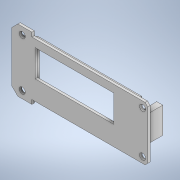
# Autodesk Inventor part: Деталь56
Saved by Autodesk Inventor 2020 (Build 240168000, 168)
## iProperties
Created: 2022-03-19
Part Number: Деталь56
Material: Типовые
Document SubType Name: Modeling
Designer: NoName
Density: 1 g/cm^3
Appearance: По умолчанию
Author: NoName
Autodesk Inventor part; units mm, degrees
ref_plane "YZ Plane" through (0, 0, 0) normal (1, 0, 0) x (0, 1, 0)
ref_plane "XZ Plane" through (0, 0, 0) normal (0, 1, 0) x (-1, 0, 0)
ref_plane "XY Plane" through (0, 0, 0) normal (0, 0, 1) x (1, 0, 0)
sketch "Эскиз1" plane through (0, 0, 0) normal (0, 0, 1) x (1, 0, 0)
  line L0 (40.25, 0.65) -> (37.25, 0.65) projected
  line L1 (37.25, 0.65) -> (37.25, -2.2) projected
  arc A0 (37.25, -2.2) -> (39.25, -4.2) centre (39.25, -2.2) ccw projected
  line L2 (39.25, -4.2) -> (39.25, -12.9) projected
  arc A1 (39.25, -12.9) -> (37.25, -14.9) centre (39.25, -14.9) ccw projected
  line L3 (37.25, -14.9) -> (37.25, -17.75) projected
  line L4 (37.25, -17.75) -> (40.25, -17.75) projected
  line L5 (40.25, -17.75) -> (41.25, -16.75) projected
  line L6 (41.25, -16.75) -> (41.25, -0.35) projected
  line L7 (41.25, -0.35) -> (40.25, 0.65) projected
  circle A2 centre (39.3375, -15.55) radius 1 projected
  circle A3 centre (39.3375, -1.55) radius 1 projected
  line L8 (2.55, -18.95) -> (2.55, -17.75) projected
  line L9 (2.55, -17.75) -> (2.55, -16.45) projected
  line L10 (0.65, -14.55) -> (2.55, -16.45) projected
  line L11 (-4.15, -14.55) -> (0.65, -14.55) projected
  line L12 (-4.15, -14.55) -> (-4.15, -16.95) projected
  line L13 (-4.15, -16.95) -> (-2.15, -18.95) projected
  line L14 (-2.15, -18.95) -> (2.55, -18.95) projected
  circle A4 centre (-0.65, -16.55) radius 1 projected
  line L15 (2.55, 0.65) -> (2.55, 1.85) projected
  line L16 (2.55, 1.85) -> (-2.15, 1.85) projected
  line L17 (-2.15, 1.85) -> (-4.15, -0.15) projected
  line L18 (-4.15, -0.15) -> (-4.15, -2.55) projected
  line L19 (0.65, -2.55) -> (-4.15, -2.55) projected
  line L20 (2.55, -0.65) -> (0.65, -2.55) projected
  line L21 (2.55, -0.65) -> (2.55, 0.65) projected
  circle A5 centre (-0.65, -0.55) radius 1 projected
  line L22 (2.55, 0.65) -> (40.25, 0.65) projected
  line L23 (40.25, -17.75) -> (2.55, -17.75) projected
  line L24 (-4.15, -14.55) -> (-4.15, -2.55) projected
  point P0 (0, 0)
extrude "Выдавливание1" add sketch "Эскиз1" along normal blind 0.8
sketch "Эскиз2" plane through (0, 0, 0.8) normal (0, 0, 1) x (1, 0, 0)
  line L0 (3.65, -11.05) -> (29.75, -11.05)
  line L1 (29.75, -11.05) -> (29.75, -2.05)
  line L2 (29.75, -2.05) -> (3.65, -2.05)
  line L3 (3.65, -2.05) -> (3.65, -11.05)
  line L4 (40.25, 0.65) -> (2.55, 0.65) projected
  line L5 (41.25, -16.75) -> (41.25, -0.35) projected
  point P0 (0, 0)
  dimension "d2" = 9
  dimension "d3" = 26.1
  dimension "d4" = 2.7
  dimension "d5" = 11.5
  constraints: 8 end point, 2 parallel, 1 horizontal, 1 perpendicular
  measures "d2" distance between parallel lines of L0 L2
  measures "d3" distance between parallel lines of L1 L3
  measures "d4" distance between parallel lines of L4 L2
  measures "d5" distance between parallel lines of L5 L1
extrude "Выдавливание2" cut sketch "Эскиз2" against normal through all
sketch "Эскиз3" plane through (0, 0, 0) normal (0, 0, -1) x (-1, 0, 0)
  line L0 (-40.25, 0.65) -> (-37.25, 0.65) projected
  line L1 (-37.25, 0.65) -> (-37.25, -2.2) projected
  arc A0 (-39.25, -4.2) -> (-37.25, -2.2) centre (-39.25, -2.2) ccw projected
  line L2 (-39.25, -4.2) -> (-39.25, -12.9) projected
  arc A1 (-37.25, -14.9) -> (-39.25, -12.9) centre (-39.25, -14.9) ccw projected
  line L3 (-37.25, -14.9) -> (-37.25, -17.75) projected
  line L4 (-37.25, -17.75) -> (-40.25, -17.75) projected
  line L5 (-40.25, -17.75) -> (-41.25, -16.75) projected
  line L6 (-41.25, -16.75) -> (-41.25, -0.35) projected
  line L7 (-41.25, -0.35) -> (-40.25, 0.65) projected
  circle A2 centre (-39.3375, -15.55) radius 1 projected
  circle A3 centre (-39.3375, -1.55) radius 1 projected
  line L8 (-2.55, 0.65) -> (-2.55, 1.85) projected
  line L9 (-2.55, 1.85) -> (2.15, 1.85) projected
  line L10 (2.15, 1.85) -> (4.15, -0.15) projected
  line L11 (4.15, -0.15) -> (4.15, -2.55) projected
  line L12 (-0.65, -2.55) -> (4.15, -2.55) projected
  line L13 (-2.55, -0.65) -> (-0.65, -2.55) projected
  line L14 (-2.55, -0.65) -> (-2.55, 0.65) projected
  circle A4 centre (0.65, -0.55) radius 1 projected
  line L15 (-2.55, -18.95) -> (-2.55, -17.75) projected
  line L16 (-2.55, -17.75) -> (-2.55, -16.45) projected
  line L17 (-0.65, -14.55) -> (-2.55, -16.45) projected
  line L18 (4.15, -14.55) -> (-0.65, -14.55) projected
  line L19 (4.15, -14.55) -> (4.15, -16.95) projected
  line L20 (4.15, -16.95) -> (2.15, -18.95) projected
  line L21 (2.15, -18.95) -> (-2.55, -18.95) projected
  circle A5 centre (0.65, -16.55) radius 1 projected
  line L22 (-2.55, -17.75) -> (-40.25, -17.75) projected
  line L23 (4.15, -2.55) -> (4.15, -14.55)
  line L24 (4.15, -0.15) -> (4.15, -16.95) projected
  line L25 (-3.25, -13.35) -> (-35.75, -13.35)
  line L26 (-35.75, -13.35) -> (-35.75, -1.45)
  line L27 (-35.75, -1.45) -> (-3.25, -1.45)
  line L28 (-3.25, -1.45) -> (-3.25, -13.35)
  line L29 (-29.75, -11.05) -> (-29.75, -2.05) projected
  line L30 (-3.65, -11.05) -> (-29.75, -11.05) projected
  line L31 (-3.65, -2.05) -> (-3.65, -11.05) projected
  line L32 (-29.75, -2.05) -> (-3.65, -2.05) projected
  line L33 (2.15, 1.85) -> (-43.25, 1.85) projected
  line L34 (-43.25, -18.95) -> (2.15, -18.95) projected
  line L35 (-37.25, -0.15) -> (-2.55, -0.15)
  line L36 (-37.25, -16.95) -> (-2.55, -16.95)
  point P0 (0, 0)
  dimension "d13" = 6
  dimension "d15" = 0.4
  dimension "d17" = 2.3
  dimension "d18" = 0.6
  dimension "d21" = 2
  dimension "d22" = 2
  constraints: 14 end point, 4 point on line, 3 perpendicular, 2 parallel, 1 collinear, 1 horizontal
  measures "d13" distance between parallel lines of L26 L29
  measures "d15" distance between parallel lines of L31 L28
  measures "d17" distance between parallel lines of L25 L30
  measures "d18" distance between parallel lines of L27 L32
  measures "d21" distance between parallel lines of L33 L35
  measures "d22" distance between parallel lines of L34 L36
extrude "Выдавливание3" add sketch "Эскиз3" along normal blind 1 contours L35 L14 L13 L12 L23 L18 L17 L16 L36 L3 A1 L2 A0 L1
sketch "Эскиз4" plane through (0, 0, -1) normal (0, 0, -1) x (-1, 0, 0)
  line L0 (-0.65, -2.55) -> (4.15, -2.55) projected
  line L1 (-2.55, -16.45) -> (-0.65, -14.55) projected
  line L2 (4.15, -2.55) -> (-0.65, -2.55)
  line L3 (-0.65, -2.55) -> (-0.65, -14.55)
  line L4 (-0.65, -14.55) -> (4.15, -14.55)
  line L5 (4.15, -14.55) -> (4.15, -2.55)
  point P0 (0, 0)
  constraints: 8 end point, 2 parallel, 1 horizontal, 1 perpendicular
extrude "Выдавливание4" add sketch "Эскиз4" along normal blind 0.4
sketch "Эскиз5" plane through (0, 0, -1) normal (0, 0, -1) x (-1, 0, 0)
  line L0 (-39.25, -4.2) -> (-39.25, -12.9) projected
  line L1 (-39.25, -4.2) -> (-37.25, -4.2)
  line L2 (-37.25, -4.2) -> (-37.25, -12.9)
  line L3 (-37.25, -12.9) -> (-39.25, -12.9)
  line L4 (-39.25, -12.9) -> (-39.25, -4.2)
  point P0 (0, 0)
  dimension "d25" = 2
  constraints: 8 end point, 2 parallel, 1 horizontal, 1 perpendicular
  measures "d25" distance between parallel lines of L0 L2
extrude "Выдавливание5" add sketch "Эскиз5" along normal blind 5
sketch "Эскиз7" plane through (0, 0, 0.8) normal (0, 0, 1) x (1, 0, 0)
  line L0 (2.55, -17.75) -> (40.25, -17.75) projected
  line L1 (2.55, -17.75) -> (2.55, -17.55)
  line L2 (2.55, -17.55) -> (40.1672, -17.55)
  line L3 (40.1672, -17.55) -> (41.05, -16.6672)
  line L4 (41.05, -16.6672) -> (41.05, -8.55)
  line L5 (41.25, -16.75) -> (41.25, -0.35) projected
  line L6 (41.25, -8.55) -> (-4.15, -8.55)
  line L7 (-4.15, -0.15) -> (-4.15, -16.95) projected
  line L8 (40.25, -17.75) -> (41.25, -16.75) projected
  line L9 (2.55, 0.45) -> (40.1672, 0.45)
  line L10 (40.1672, 0.45) -> (41.05, -0.4328)
  line L11 (41.05, -0.4328) -> (41.05, -8.55)
  line L12 (35.75, -1.45) -> (35.75, -13.35) projected
  line L13 (29.75, -11.05) -> (3.65, -11.05) projected
  line L14 (3.65, -11.05) -> (3.65, -2.05) projected
  line L15 (3.65, -2.05) -> (29.75, -2.05) projected
  line L16 (29.75, -2.05) -> (29.75, -11.05) projected
  line L17 (-4.15, -0.15) -> (-4.15, -16.95) projected
  line L18 (-4.15, -16.95) -> (-2.15, -18.95) projected
  line L19 (-2.15, -18.95) -> (2.55, -18.95) projected
  line L20 (2.55, -18.95) -> (2.55, -17.75) projected
  line L21 (2.55, -17.75) -> (40.25, -17.75) projected
  line L22 (40.25, -17.75) -> (41.25, -16.75) projected
  line L23 (41.25, -16.75) -> (41.25, -0.35) projected
  line L24 (41.25, -0.35) -> (40.25, 0.65) projected
  line L25 (40.25, 0.65) -> (2.55, 0.65) projected
  line L26 (2.55, 0.65) -> (2.55, 1.85) projected
  line L27 (2.55, 1.85) -> (-2.15, 1.85) projected
  line L28 (-2.15, 1.85) -> (-4.15, -0.15) projected
  circle A0 centre (-0.65, -16.55) radius 1 projected
  circle A1 centre (-0.65, -0.55) radius 1 projected
  circle A2 centre (39.3375, -1.55) radius 1 projected
  circle A3 centre (39.3375, -15.55) radius 1 projected
  line L29 (2.55, 0.45) -> (2.55, 0.65)
  line L30 (40.25, 0.65) -> (2.55, 0.65) projected
  line L31 (2.55, 0.65) -> (40.25, 0.65)
  line L32 (41.25, -0.35) -> (40.25, 0.65) projected
  line L33 (40.25, 0.65) -> (41.25, -0.35)
  point P0 (0, 0)
  point P1 (41.25, -0.35)
  dimension "d33" = 0.2
  dimension "d34" = 0.2
  dimension "d35" = 0.2
  constraints: 22 end point, 3 symmetric about line, 2 collinear, 2 midpoint, 2 parallel, 2 vertical, 1 perpendicular, 1 point on line
  measures "d33" distance between parallel lines of L0 L2
  measures "d34" distance between parallel lines of L5 L4
  measures "d35" distance between parallel lines of L8 L3
extrude "Выдавливание7" cut sketch "Эскиз7" against normal through all contours L1 L2 L3 L4 L6 L5 L8 L0 | L6 L11 L10 L9 L29 L25 L24 L5
